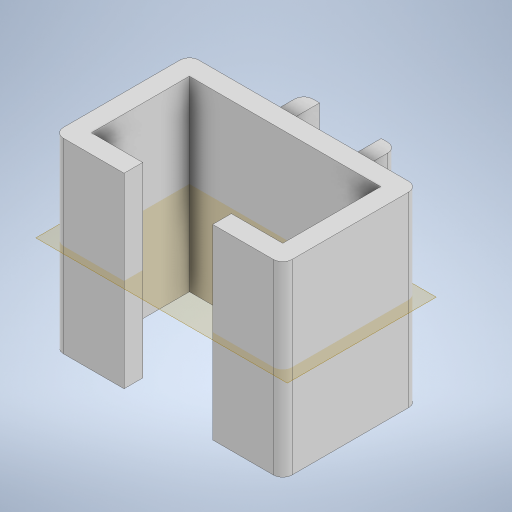
# Autodesk Inventor part: 지그1
Saved by Autodesk Inventor 2023 (Build 270158000, 158)
## iProperties
Created: 2023-08-24
Part Number: 지그1
Material: 일반
Document SubType Name: Modeling
Designer: rlatk
Density: 1 g/cm^3
Appearance: 기본값
Author: rlatk
Autodesk Inventor part; units mm, degrees
ref_plane "YZ Plane" through (0, 0, 0) normal (1, 0, 0) x (0, 1, 0)
ref_plane "XZ Plane" through (0, 0, 0) normal (0, 1, 0) x (-1, 0, 0)
ref_plane "XY Plane" through (0, 0, 0) normal (0, 0, 1) x (1, 0, 0)
sketch "스케치1" plane through (0, 0, 0) normal (0, 1, 0) x (-1, 0, 0)
  line L0 (41, 0) -> (41, -21)
  line L1 (41, -21) -> (0, -21)
  line L2 (0, -21) -> (0, 0)
  line L3 (-4, -25) -> (45, -25)
  line L4 (45, -25) -> (45, 4)
  line L5 (-4, 4) -> (-4, -25)
  line L6 (41, -21) -> (0, -21)
  line L7 (30, 0) -> (30, 4)
  line L8 (11, 0) -> (11, 4)
  line L9 (0, 0) -> (11, 0)
  line L10 (30, 0) -> (41, 0)
  line L11 (45, 4) -> (30, 4)
  line L12 (11, 4) -> (-4, 4)
  line L13 (41, 0) -> (30, 0)
  line L14 (11, 0) -> (0, 0)
  dimension "d0" = 41
  dimension "d1" = 21
  dimension "d2" = 4
  dimension "d3" = 15
  dimension "d4" = 15
  constraints: 30 end point, 8 perpendicular, 6 parallel, 2 horizontal, 1 point on line, 1 other
  measures "d0" distance of L0.end L1.end
  measures "d1" distance of L0.end L0.start
  measures "d2" distance between parallel lines of L1 L3
  measures "d3" distance between parallel lines of L4 L7
  measures "d4" distance between parallel lines of L5 L8
extrude "돌출1" add sketch "스케치1" along normal blind 40
ref_plane "작업 평면1" through (0, 20, 0) normal (0, 1, 0) x (1, 0, 0)
sketch "스케치3" plane through (0, 20, 0) normal (0, 1, 0) x (1, 0, 0)
  line L0 (-10.5, 25) -> (-10.5, 35)
  line L1 (-10.5, 35) -> (-30.5, 35)
  line L2 (-30.5, 35) -> (-30.5, 25)
  line L3 (4, 25) -> (-45, 25) projected
  line L4 (-20.5, 25) -> (-10.5, 35) construction
  line L5 (-20.5, 25) -> (-30.5, 35) construction
  point P0 (0, 0)
  dimension "d12" = 20
  constraints: 10 end point, 2 midpoint, 2 point on line, 1 parallel
  measures "d12" distance of L1.end L0.end
extrude "돌출2" add sketch "스케치3" along normal blind 15 and the other way blind 15
sketch "스케치4" plane through (-10.5, 35, -35) normal (0, 0, -1) x (-1, 0, 0)
  line L0 (20, 0) -> (20, -30) projected
  line L1 (0, 0) -> (20, 0) projected
  line L2 (0, -30) -> (0, 0) projected
  line L3 (20, -30) -> (0, -30) projected
  line L4 (0, 0) -> (20, 0) projected
  line L5 (16.6, -39.6) -> (3.4, -39.6)
  line L6 (3.4, -39.6) -> (3.4, 0)
  line L7 (3.4, 0) -> (16.6, 0)
  line L8 (16.6, 0) -> (16.6, -39.6)
  line L9 (16.6, -39.6) -> (3.4, 0) construction
  line L10 (3.4, -39.6) -> (16.6, 0) construction
  point P0 (-10.5, -35)
  point P1 (10, -19.8)
  point P2 (16.6, -30)
  point P3 (16.6, 0)
  point P4 (3.4, -30)
  point P5 (10, 0)
  dimension "d18" = 13.2
  constraints: 12 end point, 4 midpoint, 2 parallel, 1 horizontal, 1 perpendicular, 1 point on line
  measures "d18" distance of L6.end L7.end
extrude "돌출3" cut sketch "스케치4" against normal blind 10 contours L8 L3 L6 L1
fillet "모깎기1" radius 2 8 edges at (-30.5, 20, -35) (-10.5, 20, -35) (-10.5, 20, -25) (-30.5, 20, -25) (-45, 20, -25) (4, 20, -25) (4, 20, 4) (-45, 20, 4)
